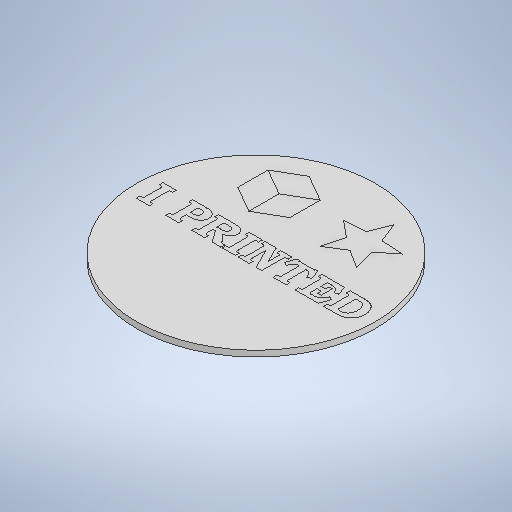
# Autodesk Inventor part: I_Printed
Saved by Autodesk Inventor 2025 (Build 290162000, 162)
## iProperties
Created: 2024-07-08
Part Number: I_Printed
Material: Generic
Document SubType Name: Modeling
Designer: ethan
Density: 1 g/cm^3
Appearance: Default
Author: ethan
Autodesk Inventor part; units mm, degrees
(part 1 of 2)
ref_plane "YZ Plane" through (0, 0, 0) normal (1, 0, 0) x (0, 1, 0)
ref_plane "XZ Plane" through (0, 0, 0) normal (0, 1, 0) x (-1, 0, 0)
ref_plane "XY Plane" through (0, 0, 0) normal (0, 0, 1) x (1, 0, 0)
sketch "Sketch2" plane through (0, 0, 0) normal (0, 1, 0) x (-1, 0, 0)
  circle A0 centre (0, 0) radius 50.8
  dimension "d2" = 101.6
  constraints: 1 centre point, 1 coincident
  measures "d2" diameter of A0
extrude "Extrusion1" add sketch "Sketch2" along normal blind 2.54
sketch "Sketch3" plane through (0, 2.54, 0) normal (0, 1, 0) x (1, 0, 0)
  line L0 (-46.0267, 6.3644) -> (46.9491, 6.3644) construction
  line L1 (46.9491, 6.3644) -> (46.9491, -11.3453) construction
  line L2 (46.9491, -11.3453) -> (-46.0267, -11.3453) construction
  line L3 (-46.0267, -11.3453) -> (-46.0267, 6.3644) construction
  line L4 (-45.4605, 5.9805) -> (-39.8942, 5.9805)
  line L5 (-39.8942, 5.9805) -> (-39.8942, 4.397)
  line L6 (-39.8942, 4.397) -> (-40.4028, 4.397)
  spline S0 degree 2 poles (-40.4028, 4.397) (-40.8443, 4.397) (-41.1322, 4.2435) (-41.2666, 3.9076) (-41.2666, 3.4277) knots 0 0 0 1 2 3 3 3
  line L7 (-41.2666, 3.4277) -> (-41.2666, -2.8871)
  spline S1 degree 2 poles (-41.2666, -2.8871) (-41.2666, -3.4053) (-41.1514, -3.7028) (-41.0171, -3.77) knots 0 0 0 1 2 2 2
  spline S2 degree 2 poles (-41.0171, -3.77) (-40.8443, -3.866) (-40.4988, -3.866) knots 0 0 0 1 1 1
  line L8 (-40.4988, -3.866) -> (-39.8942, -3.866)
  line L9 (-39.8942, -3.866) -> (-39.8942, -5.4495)
  line L10 (-39.8942, -5.4495) -> (-45.4605, -5.4495)
  line L11 (-45.4605, -5.4495) -> (-45.4605, -3.866)
  line L12 (-45.4605, -3.866) -> (-45.0094, -3.866)
  spline S3 degree 2 poles (-45.0094, -3.866) (-44.52, -3.866) (-44.232, -3.722) (-44.0881, -3.4245) (-44.0881, -2.9734) knots 0 0 0 1 2 3 3 3
  line L13 (-44.0881, -2.9734) -> (-44.0881, 3.3702)
  spline S4 degree 2 poles (-44.0881, 3.3702) (-44.0881, 3.9076) (-44.232, 4.2435) (-44.3952, 4.3299) knots 0 0 0 1 2 2 2
  spline S5 degree 2 poles (-44.3952, 4.3299) (-44.5104, 4.397) (-44.9518, 4.397) knots 0 0 0 1 1 1
  line L14 (-44.9518, 4.397) -> (-45.4605, 4.397)
  line L15 (-45.4605, 4.397) -> (-45.4605, 5.9805)
  line L16 (-32.946, 5.9805) -> (-26.9095, 5.9805)
  spline S6 degree 2 poles (-26.9095, 5.9805) (-25.7675, 5.9805) (-24.2511, 5.5103) (-23.1571, 4.5602) (-22.5717, 3.2646) (-22.5717, 2.5352) knots 0 0 0 1 2 3 4 4 4
  spline S7 degree 2 poles (-22.5717, 2.5352) (-22.5717, 1.0669) (-24.827, -0.9197) (-26.8039, -0.9197) knots 0 0 0 1 2 2 2
  line L17 (-26.8039, -0.9197) -> (-28.7521, -0.9197)
  line L18 (-28.7521, -0.9197) -> (-28.7521, -3.0598)
  spline S8 degree 2 poles (-28.7521, -3.0598) (-28.7521, -3.4533) (-28.6945, -3.5589) knots 0 0 0 1 1 1
  spline S9 degree 2 poles (-28.6945, -3.5589) (-28.6178, -3.722) (-28.3203, -3.866) (-27.9556, -3.866) knots 0 0 0 1 2 2 2
  line L19 (-27.9556, -3.866) -> (-27.3797, -3.866)
  line L20 (-27.3797, -3.866) -> (-27.3797, -5.4495)
  line L21 (-27.3797, -5.4495) -> (-32.946, -5.4495)
  line L22 (-32.946, -5.4495) -> (-32.946, -3.866)
  line L23 (-32.946, -3.866) -> (-32.5621, -3.866)
  spline S10 degree 2 poles (-32.5621, -3.866) (-32.0535, -3.866) (-31.7176, -3.722) (-31.5736, -3.3957) (-31.5736, -2.8967) knots 0 0 0 1 2 3 3 3
  line L24 (-31.5736, -2.8967) -> (-31.5736, 3.3798)
  spline S11 degree 2 poles (-31.5736, 3.3798) (-31.5736, 3.9076) (-31.708, 4.2435) (-31.9959, 4.397) (-32.399, 4.397) knots 0 0 0 1 2 3 3 3
  line L25 (-32.399, 4.397) -> (-32.946, 4.397)
  line L26 (-32.946, 4.397) -> (-32.946, 5.9805)
  line L27 (-28.7521, 4.1091) -> (-28.7521, 0.8653)
  line L28 (-28.7521, 0.8653) -> (-27.7828, 0.8653)
  spline S12 degree 2 poles (-27.7828, 0.8653) (-26.8903, 0.8653) (-26.0554, 1.23) (-25.5467, 1.9978) (-25.5467, 2.516) knots 0 0 0 1 2 3 3 3
  spline S13 degree 2 poles (-25.5467, 2.516) (-25.5467, 3.303) (-26.1513, 3.7636) knots 0 0 0 1 1 1
  spline S14 degree 2 poles (-26.1513, 3.7636) (-26.6024, 4.1091) (-27.4853, 4.1091) knots 0 0 0 1 1 1
  line L29 (-27.4853, 4.1091) -> (-28.7521, 4.1091)
  line L30 (-21.9383, 5.9805) -> (-14.8941, 5.9805)
  spline S15 degree 2 poles (-14.8941, 5.9805) (-14.2127, 5.9805) (-12.6004, 5.731) (-11.2952, 4.8961) (-10.5754, 3.6197) (-10.5754, 2.8135) knots 0 0 0 1 2 3 4 4 4
  spline S16 degree 2 poles (-10.5754, 2.8135) (-10.5754, 1.5179) (-12.4373, -0.104) (-13.7041, -0.3439) knots 0 0 0 1 2 2 2
  line L31 (-13.7041, -0.3439) -> (-11.3528, -3.079)
  line L32 (-11.3528, -3.079) -> (-11.2568, -3.2038)
  spline S17 degree 2 poles (-11.2568, -3.2038) (-11.0265, -3.4821) (-10.6426, -3.7508) (-10.2683, -3.866) (-9.9324, -3.866) knots 0 0 0 1 2 3 3 3
  line L33 (-9.9324, -3.866) -> (-9.443, -3.866)
  line L34 (-9.443, -3.866) -> (-9.443, -5.4495)
  line L35 (-9.443, -5.4495) -> (-13.109, -5.4495)
  line L36 (-13.109, -5.4495) -> (-16.7751, -0.5262)
  line L37 (-16.7751, -0.5262) -> (-17.7252, -0.5262)
  line L38 (-17.7252, -0.5262) -> (-17.7252, -2.8007)
  spline S18 degree 2 poles (-17.7252, -2.8007) (-17.7252, -3.3957) (-17.5908, -3.7124) (-17.3125, -3.866) (-16.8711, -3.866) knots 0 0 0 1 2 3 3 3
  line L39 (-16.8711, -3.866) -> (-16.3528, -3.866)
  line L40 (-16.3528, -3.866) -> (-16.3528, -5.4495)
  line L41 (-16.3528, -5.4495) -> (-21.9383, -5.4495)
  line L42 (-21.9383, -5.4495) -> (-21.9383, -3.866)
  line L43 (-21.9383, -3.866) -> (-21.4296, -3.866)
  spline S19 degree 2 poles (-21.4296, -3.866) (-21.0266, -3.866) (-20.6907, -3.6932) (-20.6043, -3.5205) knots 0 0 0 1 2 2 2
  spline S20 degree 2 poles (-20.6043, -3.5205) (-20.5659, -3.4245) (-20.5659, -2.9063) knots 0 0 0 1 1 1
  line L44 (-20.5659, -2.9063) -> (-20.5659, 3.5237)
  spline S21 degree 2 poles (-20.5659, 3.5237) (-20.5659, 3.898) (-20.6907, 4.2147) (-20.825, 4.2627) knots 0 0 0 1 2 2 2
  spline S22 degree 2 poles (-20.825, 4.2627) (-21.0266, 4.3586) (-21.2761, 4.3586) knots 0 0 0 1 1 1
  line L45 (-21.2761, 4.3586) -> (-21.5064, 4.349)
  line L46 (-21.5064, 4.349) -> (-21.9383, 4.349)
  line L47 (-21.9383, 4.349) -> (-21.9383, 5.9805)
  line L48 (-17.7252, 4.0995) -> (-17.7252, 1.1437)
  line L49 (-17.7252, 1.1437) -> (-16.0265, 1.1437)
  spline S23 degree 2 poles (-16.0265, 1.1437) (-15.0284, 1.1437) (-14.04, 1.5083) (-13.5409, 2.1993) (-13.5409, 2.6888) knots 0 0 0 1 2 3 3 3
  spline S24 degree 2 poles (-13.5409, 2.6888) (-13.5409, 3.1398) (-14.0112, 3.7924) (-14.8653, 4.0995) (-15.8442, 4.0995) knots 0 0 0 1 2 3 3 3
  line L50 (-15.8442, 4.0995) -> (-17.7252, 4.0995)
  line L51 (-8.896, 5.9805) -> (-3.3297, 5.9805)
  line L52 (-3.3297, 5.9805) -> (-3.3297, 4.397)
  line L53 (-3.3297, 4.397) -> (-3.8384, 4.397)
  spline S25 degree 2 poles (-3.8384, 4.397) (-4.2798, 4.397) (-4.5677, 4.2435) (-4.7021, 3.9076) (-4.7021, 3.4277) knots 0 0 0 1 2 3 3 3
  line L54 (-4.7021, 3.4277) -> (-4.7021, -2.8871)
  spline S26 degree 2 poles (-4.7021, -2.8871) (-4.7021, -3.4053) (-4.5869, -3.7028) (-4.4526, -3.77) knots 0 0 0 1 2 2 2
  spline S27 degree 2 poles (-4.4526, -3.77) (-4.2798, -3.866) (-3.9343, -3.866) knots 0 0 0 1 1 1
  line L55 (-3.9343, -3.866) -> (-3.3297, -3.866)
  line L56 (-3.3297, -3.866) -> (-3.3297, -5.4495)
  line L57 (-3.3297, -5.4495) -> (-8.896, -5.4495)
  line L58 (-8.896, -5.4495) -> (-8.896, -3.866)
  line L59 (-8.896, -3.866) -> (-8.4449, -3.866)
  spline S28 degree 2 poles (-8.4449, -3.866) (-7.9555, -3.866) (-7.6676, -3.722) (-7.5236, -3.4245) (-7.5236, -2.9734) knots 0 0 0 1 2 3 3 3
  line L60 (-7.5236, -2.9734) -> (-7.5236, 3.3702)
  spline S29 degree 2 poles (-7.5236, 3.3702) (-7.5236, 3.9076) (-7.6676, 4.2435) (-7.8307, 4.3299) knots 0 0 0 1 2 2 2
  spline S30 degree 2 poles (-7.8307, 4.3299) (-7.9459, 4.397) (-8.3873, 4.397) knots 0 0 0 1 1 1
  line L61 (-8.3873, 4.397) -> (-8.896, 4.397)
  line L62 (-8.896, 4.397) -> (-8.896, 5.9805)
  line L63 (-2.1013, 5.9805) -> (2.5244, 5.9805)
  line L64 (2.5244, 5.9805) -> (5.8834, -0.6894)
  line L65 (5.8834, -0.6894) -> (5.8834, 3.3893)
  spline S31 degree 2 poles (5.8834, 3.3893) (5.8834, 3.9172) (5.8258, 4.0419) knots 0 0 0 1 1 1
  spline S32 degree 2 poles (5.8258, 4.0419) (5.749, 4.2435) (5.4707, 4.397) (5.0676, 4.397) knots 0 0 0 1 2 2 2
  line L66 (5.0676, 4.397) -> (4.511, 4.397)
  line L67 (4.511, 4.397) -> (4.511, 5.9805)
  line L68 (4.511, 5.9805) -> (9.2135, 5.9805)
  line L69 (9.2135, 5.9805) -> (9.2135, 4.397)
  line L70 (9.2135, 4.397) -> (8.6953, 4.397)
  spline S33 degree 2 poles (8.6953, 4.397) (8.3018, 4.397) (7.9755, 4.2147) (7.8412, 3.9076) (7.8412, 3.3893) knots 0 0 0 1 2 3 3 3
  line L71 (7.8412, 3.3893) -> (7.8412, -5.4495)
  line L72 (7.8412, -5.4495) -> (5.4899, -5.4495)
  line L73 (5.4899, -5.4495) -> (1.248, 2.9767)
  line L74 (1.248, 2.9767) -> (1.248, -2.9159)
  spline S34 degree 2 poles (1.248, -2.9159) (1.248, -3.4245) (1.3728, -3.7028) (1.6895, -3.866) (2.0734, -3.866) knots 0 0 0 1 2 3 3 3
  line L75 (2.0734, -3.866) -> (2.6204, -3.866)
  line L76 (2.6204, -3.866) -> (2.6204, -5.4495)
  line L77 (2.6204, -5.4495) -> (-2.1013, -5.4495)
  line L78 (-2.1013, -5.4495) -> (-2.1013, -3.866)
  line L79 (-2.1013, -3.866) -> (-1.6119, -3.866)
  spline S35 degree 2 poles (-1.6119, -3.866) (-1.2088, -3.866) (-0.9113, -3.722) (-0.7289, -3.3861) (-0.7289, -3.0406) knots 0 0 0 1 2 3 3 3
  line L80 (-0.7289, -3.0406) -> (-0.7289, 3.5141)
  spline S36 degree 2 poles (-0.7289, 3.5141) (-0.7289, 3.8884) (-0.8921, 4.2435) (-1.1704, 4.397) (-1.4967, 4.397) knots 0 0 0 1 2 3 3 3
  line L81 (-1.4967, 4.397) -> (-2.1013, 4.397)
  line L82 (-2.1013, 4.397) -> (-2.1013, 5.9805)
  line L83 (11.0849, 6.3644) -> (12.1598, 6.3644)
  line L84 (12.1598, 6.3644) -> (12.275, 5.9805)
  line L85 (12.275, 5.9805) -> (18.7241, 5.9805)
  line L86 (18.7241, 5.9805) -> (18.8585, 6.3644)
  line L87 (18.8585, 6.3644) -> (19.9429, 6.3644)
  line L88 (19.9429, 6.3644) -> (21.3633, 2.3529)
  line L89 (21.3633, 2.3529) -> (19.8374, 1.825)
  spline S37 degree 2 poles (19.8374, 1.825) (19.3287, 2.8231) (19.108, 3.1302) knots 0 0 0 1 1 1
  spline S38 degree 2 poles (19.108, 3.1302) (18.6761, 3.7252) (18.1099, 4.0707) knots 0 0 0 1 1 1
  spline S39 degree 2 poles (18.1099, 4.0707) (17.6877, 4.3299) (17.2654, 4.3299) knots 0 0 0 1 1 1
  spline S40 degree 2 poles (17.2654, 4.3299) (17.0639, 4.3299) (16.9199, 4.1379) (16.9199, 3.802) knots 0 0 0 1 2 2 2
  line L90 (16.9199, 3.802) -> (16.9199, -2.7623)
  spline S41 degree 2 poles (16.9199, -2.7623) (16.9199, -3.3381) (17.0063, -3.6356) (17.1982, -3.8084) (17.5437, -3.866) (18.2923, -3.866) knots 0 0 0 1 2 3 4 4 4
  line L91 (18.2923, -3.866) -> (18.2923, -5.4495)
  line L92 (18.2923, -5.4495) -> (12.726, -5.4495)
  line L93 (12.726, -5.4495) -> (12.726, -3.866)
  line L94 (12.726, -3.866) -> (13.0619, -3.866)
  spline S42 degree 2 poles (13.0619, -3.866) (13.6185, -3.866) (13.9352, -3.722) (14.0984, -3.3765) (14.0984, -2.8199) knots 0 0 0 1 2 3 3 3
  line L95 (14.0984, -2.8199) -> (14.0984, 3.898)
  spline S43 degree 2 poles (14.0984, 3.898) (14.0984, 4.1859) (13.964, 4.3299) (13.7529, 4.3299) knots 0 0 0 1 2 2 2
  spline S44 degree 2 poles (13.7529, 4.3299) (13.3306, 4.3299) (12.275, 3.6869) (11.8719, 3.111) knots 0 0 0 1 2 2 2
  spline S45 degree 2 poles (11.8719, 3.111) (11.6991, 2.8807) (11.1713, 1.825) knots 0 0 0 1 1 1
  line L96 (11.1713, 1.825) -> (9.6742, 2.3529)
  line L97 (9.6742, 2.3529) -> (11.0849, 6.3644)
  line L98 (22.0447, 5.9805) -> (31.5841, 5.9805)
  line L99 (31.5841, 5.9805) -> (32.8893, 2.3625)
  line L100 (32.8893, 2.3625) -> (31.4017, 1.825)
  spline S46 degree 2 poles (31.4017, 1.825) (31.0275, 2.7176) (30.0198, 3.7924) (28.801, 4.1475) (27.9852, 4.1475) knots 0 0 0 1 2 3 3 3
  line L101 (27.9852, 4.1475) -> (26.2386, 4.1475)
  line L102 (26.2386, 4.1475) -> (26.2386, 1.2972)
  line L103 (26.2386, 1.2972) -> (26.8144, 1.2972)
  spline S47 degree 2 poles (26.8144, 1.2972) (27.4574, 1.2972) (27.9084, 1.4891) (28.11, 1.8826) (28.11, 2.4872) knots 0 0 0 1 2 3 3 3
  line L104 (28.11, 2.4872) -> (28.11, 2.9191)
  line L105 (28.11, 2.9191) -> (29.5687, 2.9191)
  line L106 (29.5687, 2.9191) -> (29.5687, -1.9178)
  line L107 (29.5687, -1.9178) -> (28.11, -1.9178)
  line L108 (28.11, -1.9178) -> (28.11, -1.4283)
  spline S48 degree 2 poles (28.11, -1.4283) (28.11, -0.9197) (27.87, -0.459) (27.4574, -0.2959) (26.7568, -0.2959) knots 0 0 0 1 2 3 3 3
  line L109 (26.7568, -0.2959) -> (26.2386, -0.2959)
  line L110 (26.2386, -0.2959) -> (26.2386, -2.9159)
  spline S49 degree 2 poles (26.2386, -2.9159) (26.2386, -3.3381) (26.3249, -3.5205) (26.5553, -3.6164) (26.9487, -3.6164) knots 0 0 0 1 2 3 3 3
  line L111 (26.9487, -3.6164) -> (27.9084, -3.6164)
  spline S50 degree 2 poles (27.9084, -3.6164) (28.9833, -3.6164) (30.4612, -3.0022) (31.6225, -1.6299) (31.9296, -0.6894) knots 0 0 0 1 2 3 3 3
  line L112 (31.9296, -0.6894) -> (33.4267, -1.198)
  line L113 (33.4267, -1.198) -> (31.9296, -5.4495)
  line L114 (31.9296, -5.4495) -> (22.0447, -5.4495)
  line L115 (22.0447, -5.4495) -> (22.0447, -3.866)
  line L116 (22.0447, -3.866) -> (22.3326, -3.866)
  spline S51 degree 2 poles (22.3326, -3.866) (22.8988, -3.866) (23.2923, -3.7028) (23.3787, -3.5013) knots 0 0 0 1 2 2 2
  spline S52 degree 2 poles (23.3787, -3.5013) (23.4171, -3.3765) (23.4171, -2.8007) knots 0 0 0 1 1 1
  line L117 (23.4171, -2.8007) -> (23.4171, 3.4181)
  spline S53 degree 2 poles (23.4171, 3.4181) (23.4171, 3.9268) (23.2827, 4.2435) (22.9852, 4.397) (22.5533, 4.397) knots 0 0 0 1 2 3 3 3
  line L118 (22.5533, 4.397) -> (22.0447, 4.397)
  line L119 (22.0447, 4.397) -> (22.0447, 5.9805)
  line L120 (34.0985, 5.9805) -> (40.087, 5.9805)
  spline S54 degree 2 poles (40.087, 5.9805) (42.1312, 5.9805) (44.54, 4.6849) (45.9699, 2.1417) (45.9699, 0.3663) knots 0 0 0 1 2 3 3 3
  spline S55 degree 2 poles (45.9699, 0.3663) (45.9699, -0.8717) (45.2406, -2.8199) (43.801, -4.3842) (42.9757, -4.7777) knots 0 0 0 1 2 3 3 3
  spline S56 degree 2 poles (42.9757, -4.7777) (42.3519, -5.0752) (40.0582, -5.4495) (39.3768, -5.4495) knots 0 0 0 1 2 2 2
  line L121 (39.3768, -5.4495) -> (34.0985, -5.4495)
  line L122 (34.0985, -5.4495) -> (34.0985, -3.866)
  line L123 (34.0985, -3.866) -> (34.492, -3.866)
  spline S57 degree 2 poles (34.492, -3.866) (34.991, -3.866) (35.3077, -3.7028) (35.4037, -3.5013) knots 0 0 0 1 2 2 2
  spline S58 degree 2 poles (35.4037, -3.5013) (35.4709, -3.3477) (35.4709, -2.8295) knots 0 0 0 1 1 1
  line L124 (35.4709, -2.8295) -> (35.4709, 3.4181)
  spline S59 degree 2 poles (35.4709, 3.4181) (35.4709, 3.9364) (35.3269, 4.2435) (35.0102, 4.397) (34.492, 4.397) knots 0 0 0 1 2 3 3 3
  line L125 (34.492, 4.397) -> (34.0985, 4.397)
  line L126 (34.0985, 4.397) -> (34.0985, 5.9805)
  line L127 (38.2828, 4.1475) -> (38.2828, -2.9639)
  spline S60 degree 2 poles (38.2828, -2.9639) (38.2828, -3.3189) (38.3212, -3.4053) knots 0 0 0 1 1 1
  spline S61 degree 2 poles (38.3212, -3.4053) (38.3883, -3.5301) (38.6475, -3.6164) (39.1273, -3.6164) knots 0 0 0 1 2 2 2
  spline S62 degree 2 poles (39.1273, -3.6164) (40.4709, -3.6164) (41.9872, -2.7911) (42.9181, -0.9581) (42.9181, 0.2991) knots 0 0 0 1 2 3 3 3
  spline S63 degree 2 poles (42.9181, 0.2991) (42.9181, 1.5467) (42.0448, 3.3893) (40.7492, 4.1475) (39.54, 4.1475) knots 0 0 0 1 2 3 3 3
  line L128 (39.54, 4.1475) -> (38.2828, 4.1475)
  point P0 (0, 0)
  constraints: 2 other
extrude "Extrusion2" cut sketch "Sketch3" against normal blind 10.4775
sketch "Sketch4" plane through (0, 2.54, 0) normal (0, 1, 0) x (1, 0, 0)
  circle A0 centre (0, 0) radius 50.8 projected
  line L0 (22.0447, 4.397) -> (22.0447, 5.9805) projected
  line L1 (22.0447, 5.9805) -> (31.5841, 5.9805) projected
  line L2 (31.5841, 5.9805) -> (32.8893, 2.3625) projected
  line L3 (32.8893, 2.3625) -> (31.4017, 1.825) projected
  spline S0 degree 2 poles (31.4017, 1.825) (31.0275, 2.7176) (30.0198, 3.7924) (28.801, 4.1475) (27.9852, 4.1475) knots 0 0 0 0.333333 0.666667 1 1 1 projected
  line L4 (27.9852, 4.1475) -> (26.2386, 4.1475) projected
  line L5 (26.2386, 4.1475) -> (26.2386, 1.2972) projected
  line L6 (26.2386, 1.2972) -> (26.8144, 1.2972) projected
  spline S1 degree 2 poles (26.8144, 1.2972) (27.4574, 1.2972) (27.9084, 1.4891) (28.11, 1.8826) (28.11, 2.4872) knots 0 0 0 0.333333 0.666667 1 1 1 projected
  line L7 (28.11, 2.4872) -> (28.11, 2.9191) projected
  line L8 (28.11, 2.9191) -> (29.5687, 2.9191) projected
  line L9 (29.5687, 2.9191) -> (29.5687, -1.9178) projected
  line L10 (29.5687, -1.9178) -> (28.11, -1.9178) projected
  line L11 (28.11, -1.9178) -> (28.11, -1.4283) projected
  spline S2 degree 2 poles (28.11, -1.4283) (28.11, -0.9197) (27.87, -0.459) (27.4574, -0.2959) (26.7568, -0.2959) knots 0 0 0 0.333333 0.666667 1 1 1 projected
  line L12 (26.7568, -0.2959) -> (26.2386, -0.2959) projected
  line L13 (26.2386, -0.2959) -> (26.2386, -2.9159) projected
  spline S3 degree 2 poles (26.2386, -2.9159) (26.2386, -3.3381) (26.3249, -3.5205) (26.5553, -3.6164) (26.9487, -3.6164) knots 0 0 0 0.333333 0.666667 1 1 1 projected
  line L14 (26.9487, -3.6164) -> (27.9084, -3.6164) projected
  spline S4 degree 2 poles (27.9084, -3.6164) (28.9833, -3.6164) (30.4612, -3.0022) (31.6225, -1.6299) (31.9296, -0.6894) knots 0 0 0 0.333333 0.666667 1 1 1 projected
  line L15 (31.9296, -0.6894) -> (33.4267, -1.198) projected
  line L16 (33.4267, -1.198) -> (31.9296, -5.4495) projected
  line L17 (31.9296, -5.4495) -> (22.0447, -5.4495) projected
  line L18 (22.0447, -5.4495) -> (22.0447, -3.866) projected
  line L19 (22.0447, -3.866) -> (22.3326, -3.866) projected
  spline S5 degree 2 poles (22.3326, -3.866) (22.8988, -3.866) (23.2923, -3.7028) (23.3787, -3.5013) knots 0 0 0 0.5 1 1 1 projected
  spline S6 degree 2 poles (23.3787, -3.5013) (23.4171, -3.3765) (23.4171, -2.8007) knots 0 0 0 1 1 1 projected
  line L20 (23.4171, -2.8007) -> (23.4171, 3.4181) projected
  spline S7 degree 2 poles (23.4171, 3.4181) (23.4171, 3.9268) (23.2827, 4.2435) (22.9852, 4.397) (22.5533, 4.397) knots 0 0 0 0.333333 0.666667 1 1 1 projected
  line L21 (22.5533, 4.397) -> (22.0447, 4.397) projected
  line L22 (-2.1013, 4.397) -> (-2.1013, 5.9805) projected
  line L23 (-2.1013, 5.9805) -> (2.5244, 5.9805) projected
  line L24 (2.5244, 5.9805) -> (5.8834, -0.6894) projected
  line L25 (5.8834, -0.6894) -> (5.8834, 3.3893) projected
  spline S8 degree 2 poles (5.8834, 3.3893) (5.8834, 3.9172) (5.8258, 4.0419) knots 0 0 0 1 1 1 projected
  spline S9 degree 2 poles (5.8258, 4.0419) (5.749, 4.2435) (5.4707, 4.397) (5.0676, 4.397) knots 0 0 0 0.5 1 1 1 projected
  line L26 (5.0676, 4.397) -> (4.511, 4.397) projected
  line L27 (4.511, 4.397) -> (4.511, 5.9805) projected
  line L28 (4.511, 5.9805) -> (9.2135, 5.9805) projected
  line L29 (9.2135, 5.9805) -> (9.2135, 4.397) projected
  line L30 (9.2135, 4.397) -> (8.6953, 4.397) projected
  spline S10 degree 2 poles (8.6953, 4.397) (8.3018, 4.397) (7.9755, 4.2147) (7.8412, 3.9076) (7.8412, 3.3893) knots 0 0 0 0.333333 0.666667 1 1 1 projected
  line L31 (7.8412, 3.3893) -> (7.8412, -5.4495) projected
  line L32 (7.8412, -5.4495) -> (5.4899, -5.4495) projected
  line L33 (5.4899, -5.4495) -> (1.248, 2.9767) projected
  line L34 (1.248, 2.9767) -> (1.248, -2.9159) projected
  spline S11 degree 2 poles (1.248, -2.9159) (1.248, -3.4245) (1.3728, -3.7028) (1.6895, -3.866) (2.0734, -3.866) knots 0 0 0 0.333333 0.666667 1 1 1 projected
  line L35 (2.0734, -3.866) -> (2.6204, -3.866) projected
  line L36 (2.6204, -3.866) -> (2.6204, -5.4495) projected
  line L37 (2.6204, -5.4495) -> (-2.1013, -5.4495) projected
  line L38 (-2.1013, -5.4495) -> (-2.1013, -3.866) projected
  line L39 (-2.1013, -3.866) -> (-1.6119, -3.866) projected
  spline S12 degree 2 poles (-1.6119, -3.866) (-1.2088, -3.866) (-0.9113, -3.722) (-0.7289, -3.3861) (-0.7289, -3.0406) knots 0 0 0 0.333333 0.666667 1 1 1 projected
  line L40 (-0.7289, -3.0406) -> (-0.7289, 3.5141) projected
  spline S13 degree 2 poles (-0.7289, 3.5141) (-0.7289, 3.8884) (-0.8921, 4.2435) (-1.1704, 4.397) (-1.4967, 4.397) knots 0 0 0 0.333333 0.666667 1 1 1 projected
  line L41 (-1.4967, 4.397) -> (-2.1013, 4.397) projected
  line L42 (-45.4605, 4.397) -> (-45.4605, 5.9805) projected
  line L43 (-45.4605, 5.9805) -> (-39.8942, 5.9805) projected
  line L44 (-39.8942, 5.9805) -> (-39.8942, 4.397) projected
  line L45 (-39.8942, 4.397) -> (-40.4028, 4.397) projected
  spline S14 degree 2 poles (-40.4028, 4.397) (-40.8443, 4.397) (-41.1322, 4.2435) (-41.2666, 3.9076) (-41.2666, 3.4277) knots 0 0 0 0.333333 0.666667 1 1 1 projected
  line L46 (-41.2666, 3.4277) -> (-41.2666, -2.8871) projected
  spline S15 degree 2 poles (-41.2666, -2.8871) (-41.2666, -3.4053) (-41.1514, -3.7028) (-41.0171, -3.77) knots 0 0 0 0.5 1 1 1 projected
  spline S16 degree 2 poles (-41.0171, -3.77) (-40.8443, -3.866) (-40.4988, -3.866) knots 0 0 0 1 1 1 projected
  line L47 (-40.4988, -3.866) -> (-39.8942, -3.866) projected
  line L48 (-39.8942, -3.866) -> (-39.8942, -5.4495) projected
  line L49 (-39.8942, -5.4495) -> (-45.4605, -5.4495) projected
  line L50 (-45.4605, -5.4495) -> (-45.4605, -3.866) projected
  line L51 (-45.4605, -3.866) -> (-45.0094, -3.866) projected
  spline S17 degree 2 poles (-45.0094, -3.866) (-44.52, -3.866) (-44.232, -3.722) (-44.0881, -3.4245) (-44.0881, -2.9734) knots 0 0 0 0.333333 0.666667 1 1 1 projected
  line L52 (-44.0881, -2.9734) -> (-44.0881, 3.3702) projected
  spline S18 degree 2 poles (-44.0881, 3.3702) (-44.0881, 3.9076) (-44.232, 4.2435) (-44.3952, 4.3299) knots 0 0 0 0.5 1 1 1 projected
  spline S19 degree 2 poles (-44.3952, 4.3299) (-44.5104, 4.397) (-44.9518, 4.397) knots 0 0 0 1 1 1 projected
  line L53 (-44.9518, 4.397) -> (-45.4605, 4.397) projected
  line L54 (-32.946, 4.397) -> (-32.946, 5.9805) projected
  line L55 (-32.946, 5.9805) -> (-26.9095, 5.9805) projected
  spline S20 degree 2 poles (-26.9095, 5.9805) (-25.7675, 5.9805) (-24.2511, 5.5103) (-23.1571, 4.5602) (-22.5717, 3.2646) (-22.5717, 2.5352) knots 0 0 0 0.25 0.5 0.75 1 1 1 projected
  spline S21 degree 2 poles (-22.5717, 2.5352) (-22.5717, 1.0669) (-24.827, -0.9197) (-26.8039, -0.9197) knots 0 0 0 0.5 1 1 1 projected
  line L56 (-26.8039, -0.9197) -> (-28.7521, -0.9197) projected
  line L57 (-28.7521, -0.9197) -> (-28.7521, -3.0598) projected
  spline S22 degree 2 poles (-28.7521, -3.0598) (-28.7521, -3.4533) (-28.6945, -3.5589) knots 0 0 0 1 1 1 projected
  spline S23 degree 2 poles (-28.6945, -3.5589) (-28.6178, -3.722) (-28.3203, -3.866) (-27.9556, -3.866) knots 0 0 0 0.5 1 1 1 projected
  line L58 (-27.9556, -3.866) -> (-27.3797, -3.866) projected
  line L59 (-27.3797, -3.866) -> (-27.3797, -5.4495) projected
  line L60 (-27.3797, -5.4495) -> (-32.946, -5.4495) projected
  line L61 (-32.946, -5.4495) -> (-32.946, -3.866) projected
  line L62 (-32.946, -3.866) -> (-32.5621, -3.866) projected
  spline S24 degree 2 poles (-32.5621, -3.866) (-32.0535, -3.866) (-31.7176, -3.722) (-31.5736, -3.3957) (-31.5736, -2.8967) knots 0 0 0 0.333333 0.666667 1 1 1 projected
  line L63 (-31.5736, -2.8967) -> (-31.5736, 3.3798) projected
  spline S25 degree 2 poles (-31.5736, 3.3798) (-31.5736, 3.9076) (-31.708, 4.2435) (-31.9959, 4.397) (-32.399, 4.397) knots 0 0 0 0.333333 0.666667 1 1 1 projected
  line L64 (-32.399, 4.397) -> (-32.946, 4.397) projected
  line L65 (-21.9383, 4.349) -> (-21.9383, 5.9805) projected
  line L66 (-21.9383, 5.9805) -> (-14.8941, 5.9805) projected
  spline S26 degree 2 poles (-14.8941, 5.9805) (-14.2127, 5.9805) (-12.6004, 5.731) (-11.2952, 4.8961) (-10.5754, 3.6197) (-10.5754, 2.8135) knots 0 0 0 0.25 0.5 0.75 1 1 1 projected
  spline S27 degree 2 poles (-10.5754, 2.8135) (-10.5754, 1.5179) (-12.4373, -0.104) (-13.7041, -0.3439) knots 0 0 0 0.5 1 1 1 projected
  line L67 (-13.7041, -0.3439) -> (-11.3528, -3.079) projected
  line L68 (-11.3528, -3.079) -> (-11.2568, -3.2038) projected
  spline S28 degree 2 poles (-11.2568, -3.2038) (-11.0265, -3.4821) (-10.6426, -3.7508) (-10.2683, -3.866) (-9.9324, -3.866) knots 0 0 0 0.333333 0.666667 1 1 1 projected
  line L69 (-9.9324, -3.866) -> (-9.443, -3.866) projected
  line L70 (-9.443, -3.866) -> (-9.443, -5.4495) projected
  line L71 (-9.443, -5.4495) -> (-13.109, -5.4495) projected
  line L72 (-13.109, -5.4495) -> (-16.7751, -0.5262) projected
  line L73 (-16.7751, -0.5262) -> (-17.7252, -0.5262) projected
  line L74 (-17.7252, -0.5262) -> (-17.7252, -2.8007) projected
  spline S29 degree 2 poles (-17.7252, -2.8007) (-17.7252, -3.3957) (-17.5908, -3.7124) (-17.3125, -3.866) (-16.8711, -3.866) knots 0 0 0 0.333333 0.666667 1 1 1 projected
  line L75 (-16.8711, -3.866) -> (-16.3528, -3.866) projected
  line L76 (-16.3528, -3.866) -> (-16.3528, -5.4495) projected
  line L77 (-16.3528, -5.4495) -> (-21.9383, -5.4495) projected
  line L78 (-21.9383, -5.4495) -> (-21.9383, -3.866) projected
  line L79 (-21.9383, -3.866) -> (-21.4296, -3.866) projected
  spline S30 degree 2 poles (-21.4296, -3.866) (-21.0266, -3.866) (-20.6907, -3.6932) (-20.6043, -3.5205) knots 0 0 0 0.5 1 1 1 projected
  spline S31 degree 2 poles (-20.6043, -3.5205) (-20.5659, -3.4245) (-20.5659, -2.9063) knots 0 0 0 1 1 1 projected
  line L80 (-20.5659, -2.9063) -> (-20.5659, 3.5237) projected
  spline S32 degree 2 poles (-20.5659, 3.5237) (-20.5659, 3.898) (-20.6907, 4.2147) (-20.825, 4.2627) knots 0 0 0 0.5 1 1 1 projected
  spline S33 degree 2 poles (-20.825, 4.2627) (-21.0266, 4.3586) (-21.2761, 4.3586) knots 0 0 0 1 1 1 projected
  line L81 (-21.2761, 4.3586) -> (-21.5064, 4.349) projected
  line L82 (-21.5064, 4.349) -> (-21.9383, 4.349) projected
  line L83 (-8.896, 4.397) -> (-8.896, 5.9805) projected
  line L84 (-8.896, 5.9805) -> (-3.3297, 5.9805) projected
  line L85 (-3.3297, 5.9805) -> (-3.3297, 4.397) projected
  line L86 (-3.3297, 4.397) -> (-3.8384, 4.397) projected
  spline S34 degree 2 poles (-3.8384, 4.397) (-4.2798, 4.397) (-4.5677, 4.2435) (-4.7021, 3.9076) (-4.7021, 3.4277) knots 0 0 0 0.333333 0.666667 1 1 1 projected
  line L87 (-4.7021, 3.4277) -> (-4.7021, -2.8871) projected
  spline S35 degree 2 poles (-4.7021, -2.8871) (-4.7021, -3.4053) (-4.5869, -3.7028) (-4.4526, -3.77) knots 0 0 0 0.5 1 1 1 projected
  spline S36 degree 2 poles (-4.4526, -3.77) (-4.2798, -3.866) (-3.9343, -3.866) knots 0 0 0 1 1 1 projected
  line L88 (-3.9343, -3.866) -> (-3.3297, -3.866) projected
  line L89 (-3.3297, -3.866) -> (-3.3297, -5.4495) projected
  line L90 (-3.3297, -5.4495) -> (-8.896, -5.4495) projected
  line L91 (-8.896, -5.4495) -> (-8.896, -3.866) projected
  line L92 (-8.896, -3.866) -> (-8.4449, -3.866) projected
  spline S37 degree 2 poles (-8.4449, -3.866) (-7.9555, -3.866) (-7.6676, -3.722) (-7.5236, -3.4245) (-7.5236, -2.9734) knots 0 0 0 0.333333 0.666667 1 1 1 projected
  line L93 (-7.5236, -2.9734) -> (-7.5236, 3.3702) projected
  spline S38 degree 2 poles (-7.5236, 3.3702) (-7.5236, 3.9076) (-7.6676, 4.2435) (-7.8307, 4.3299) knots 0 0 0 0.5 1 1 1 projected
  spline S39 degree 2 poles (-7.8307, 4.3299) (-7.9459, 4.397) (-8.3873, 4.397) knots 0 0 0 1 1 1 projected
  line L94 (-8.3873, 4.397) -> (-8.896, 4.397) projected
  line L95 (9.6742, 2.3529) -> (11.0849, 6.3644) projected
  line L96 (11.0849, 6.3644) -> (12.1598, 6.3644) projected
  line L97 (12.1598, 6.3644) -> (12.275, 5.9805) projected
  line L98 (12.275, 5.9805) -> (18.7241, 5.9805) projected
  line L99 (18.7241, 5.9805) -> (18.8585, 6.3644) projected
  line L100 (18.8585, 6.3644) -> (19.9429, 6.3644) projected
  line L101 (19.9429, 6.3644) -> (21.3633, 2.3529) projected
  line L102 (21.3633, 2.3529) -> (19.8374, 1.825) projected
  spline S40 degree 2 poles (19.8374, 1.825) (19.3287, 2.8231) (19.108, 3.1302) knots 0 0 0 1 1 1 projected
  spline S41 degree 2 poles (19.108, 3.1302) (18.6761, 3.7252) (18.1099, 4.0707) knots 0 0 0 1 1 1 projected
  spline S42 degree 2 poles (18.1099, 4.0707) (17.6877, 4.3299) (17.2654, 4.3299) knots 0 0 0 1 1 1 projected
  spline S43 degree 2 poles (17.2654, 4.3299) (17.0639, 4.3299) (16.9199, 4.1379) (16.9199, 3.802) knots 0 0 0 0.5 1 1 1 projected
  line L103 (16.9199, 3.802) -> (16.9199, -2.7623) projected
  spline S44 degree 2 poles (16.9199, -2.7623) (16.9199, -3.3381) (17.0063, -3.6356) (17.1982, -3.8084) (17.5437, -3.866) (18.2923, -3.866) knots 0 0 0 0.25 0.5 0.75 1 1 1 projected
  line L104 (18.2923, -3.866) -> (18.2923, -5.4495) projected
  line L105 (18.2923, -5.4495) -> (12.726, -5.4495) projected
  line L106 (12.726, -5.4495) -> (12.726, -3.866) projected
  line L107 (12.726, -3.866) -> (13.0619, -3.866) projected
  spline S45 degree 2 poles (13.0619, -3.866) (13.6185, -3.866) (13.9352, -3.722) (14.0984, -3.3765) (14.0984, -2.8199) knots 0 0 0 0.333333 0.666667 1 1 1 projected
  line L108 (14.0984, -2.8199) -> (14.0984, 3.898) projected
  spline S46 degree 2 poles (14.0984, 3.898) (14.0984, 4.1859) (13.964, 4.3299) (13.7529, 4.3299) knots 0 0 0 0.5 1 1 1 projected
  spline S47 degree 2 poles (13.7529, 4.3299) (13.3306, 4.3299) (12.275, 3.6869) (11.8719, 3.111) knots 0 0 0 0.5 1 1 1 projected
  spline S48 degree 2 poles (11.8719, 3.111) (11.6991, 2.8807) (11.1713, 1.825) knots 0 0 0 1 1 1 projected
  line L109 (11.1713, 1.825) -> (9.6742, 2.3529) projected
  line L110 (34.0985, 4.397) -> (34.0985, 5.9805) projected
  line L111 (34.0985, 5.9805) -> (40.087, 5.9805) projected
  spline S49 degree 2 poles (40.087, 5.9805) (42.1312, 5.9805) (44.54, 4.6849) (45.9699, 2.1417) (45.9699, 0.3663) knots 0 0 0 0.333333 0.666667 1 1 1 projected
  spline S50 degree 2 poles (45.9699, 0.3663) (45.9699, -0.8717) (45.2406, -2.8199) (43.801, -4.3842) (42.9757, -4.7777) knots 0 0 0 0.333333 0.666667 1 1 1 projected
  spline S51 degree 2 poles (42.9757, -4.7777) (42.3519, -5.0752) (40.0582, -5.4495) (39.3768, -5.4495) knots 0 0 0 0.5 1 1 1 projected
  line L112 (39.3768, -5.4495) -> (34.0985, -5.4495) projected
  line L113 (34.0985, -5.4495) -> (34.0985, -3.866) projected
  line L114 (34.0985, -3.866) -> (34.492, -3.866) projected
  spline S52 degree 2 poles (34.492, -3.866) (34.991, -3.866) (35.3077, -3.7028) (35.4037, -3.5013) knots 0 0 0 0.5 1 1 1 projected
  spline S53 degree 2 poles (35.4037, -3.5013) (35.4709, -3.3477) (35.4709, -2.8295) knots 0 0 0 1 1 1 projected
  line L115 (35.4709, -2.8295) -> (35.4709, 3.4181) projected
  spline S54 degree 2 poles (35.4709, 3.4181) (35.4709, 3.9364) (35.3269, 4.2435) (35.0102, 4.397) (34.492, 4.397) knots 0 0 0 0.333333 0.666667 1 1 1 projected
  line L116 (34.492, 4.397) -> (34.0985, 4.397) projected
  line L117 (-28.7521, 0.8653) -> (-27.7828, 0.8653) projected
  spline S55 degree 2 poles (-27.7828, 0.8653) (-26.8903, 0.8653) (-26.0554, 1.23) (-25.5467, 1.9978) (-25.5467, 2.516) knots 0 0 0 0.333333 0.666667 1 1 1 projected
  spline S56 degree 2 poles (-25.5467, 2.516) (-25.5467, 3.303) (-26.1513, 3.7636) knots 0 0 0 1 1 1 projected
  spline S57 degree 2 poles (-26.1513, 3.7636) (-26.6024, 4.1091) (-27.4853, 4.1091) knots 0 0 0 1 1 1 projected
  line L118 (-27.4853, 4.1091) -> (-28.7521, 4.1091) projected
  line L119 (-28.7521, 4.1091) -> (-28.7521, 0.8653) projected
  line L120 (-17.7252, 1.1437) -> (-16.0265, 1.1437) projected
  spline S58 degree 2 poles (-16.0265, 1.1437) (-15.0284, 1.1437) (-14.04, 1.5083) (-13.5409, 2.1993) (-13.5409, 2.6888) knots 0 0 0 0.333333 0.666667 1 1 1 projected
  spline S59 degree 2 poles (-13.5409, 2.6888) (-13.5409, 3.1398) (-14.0112, 3.7924) (-14.8653, 4.0995) (-15.8442, 4.0995) knots 0 0 0 0.333333 0.666667 1 1 1 projected
  line L121 (-15.8442, 4.0995) -> (-17.7252, 4.0995) projected
  line L122 (-17.7252, 4.0995) -> (-17.7252, 1.1437) projected
  spline S60 degree 2 poles (38.2828, -2.9639) (38.2828, -3.3189) (38.3212, -3.4053) knots 0 0 0 1 1 1 projected
  spline S61 degree 2 poles (38.3212, -3.4053) (38.3883, -3.5301) (38.6475, -3.6164) (39.1273, -3.6164) knots 0 0 0 0.5 1 1 1 projected
  spline S62 degree 2 poles (39.1273, -3.6164) (40.4709, -3.6164) (41.9872, -2.7911) (42.9181, -0.9581) (42.9181, 0.2991) knots 0 0 0 0.333333 0.666667 1 1 1 projected
  spline S63 degree 2 poles (42.9181, 0.2991) (42.9181, 1.5467) (42.0448, 3.3893) (40.7492, 4.1475) (39.54, 4.1475) knots 0 0 0 0.333333 0.666667 1 1 1 projected
  line L123 (39.54, 4.1475) -> (38.2828, 4.1475) projected
  line L124 (38.2828, 4.1475) -> (38.2828, -2.9639) projected
  constraints: 64 other
extrude "Extrusion3" add sketch "Sketch4" against normal blind 2.54 separate body contours L0 L1 L2 L3 S0 L4 L5 L6 S1 L7 L8 L9 L10 L11 S2 L12 L13 S3 L14 S4 L15 L16 L17 L18 L19 S5 S6 L20 S7 L21 | L22 L23 L24 L25 S8 S9 L26 L27 L28 L29 L30 S10 L31 L32 L33 L34 S11 L35 L36 L37 L38 L39 S12 L40 S13 L41 | L42 L43 L44 L45 S14 L46 S15 S16 L47 L48 L49 L50 L51 S17 L52 S18 S19 L53 | L54 L55 S20 S21 L56 L57 S22 S23 L58 L59 L60 L61 L62 S24 L63 S25 L64 | L65 L66 S26 S27 L67 L68 S28 L69 L70 L71 L72 L73 L74 S29 L75 L76 L77 L78 L79 S30 S31 L80 S32 S33 L81 L82 | L83 L84 L85 L86 S34 L87 S35 S36 L88 L89 L90 L91 L92 S37 L93 S38 S39 L94 | L95 L96 L97 L98 L99 L100 L101 L102 S40 S41 S42 S43 L103 S44 L104 L105 L106 L107 S45 L108 S46 S47 S48 L109 | L110 L111 S49 S50 S51 L112 L113 L114 S52 S53 L115 S54 L116
sketch "Sketch5" plane through (0, 2.54, 0) normal (0, 1, 0) x (1, 0, 0)
  line L0 (-16.7308, 39.3139) -> (-5.6361, 32.9084)
  line L1 (-5.6361, 32.9084) -> (-5.6361, 20.0974)
  line L2 (-5.6361, 20.0974) -> (-16.7308, 13.6918)
  line L3 (-16.7308, 13.6918) -> (-27.8255, 20.0974)
  line L4 (-27.8255, 20.0974) -> (-27.8255, 32.9084)
  line L5 (-27.8255, 32.9084) -> (-16.7308, 39.3139)
  line L6 (22.4402, 31.1118) -> (19.0916, 39.5891)
  line L7 (22.4402, 31.1118) -> (31.5374, 30.5468)
  line L8 (24.5097, 24.7424) -> (31.5374, 30.5468)
  line L9 (24.5097, 24.7424) -> (26.7836, 15.9159)
  line L10 (26.7836, 15.9159) -> (19.0916, 20.806)
  line L11 (19.0916, 20.806) -> (11.3997, 15.9159)
  line L12 (13.6736, 24.7424) -> (11.3997, 15.9159)
  line L13 (13.6736, 24.7424) -> (6.6459, 30.5468)
  line L14 (15.7431, 31.1118) -> (6.6459, 30.5468)
  line L15 (15.7431, 31.1118) -> (19.0916, 39.5891)
  line L16 (6.6459, 30.5468) -> (8.6061, 31.9709)
  line L17 (17.1314, 38.165) -> (19.0916, 39.5891)
  line L18 (19.0916, 39.5891) -> (23.0914, 36.6832)
  line L19 (29.5772, 31.9709) -> (31.5374, 30.5468)
  line L20 (31.5374, 30.5468) -> (30.7887, 28.2424)
  line L21 (27.5323, 18.2202) -> (26.7836, 15.9159)
  line L22 (26.7836, 15.9159) -> (23.7959, 15.9159)
  line L23 (13.8227, 15.9159) -> (11.3997, 15.9159)
  line L24 (11.3997, 15.9159) -> (10.651, 18.2202)
  line L25 (8.5374, 24.7254) -> (6.6459, 30.5468)
  point P0 (0, 0)
  point P1 (-16.7308, 26.5029)
  point P2 (19.0916, 26.5029)
  point P3 (19.0916, 26.5029)
  constraints: 52 end point, 10 point on line, 2 horizontal, 1 coincident, 1 vertical, 25 other
extrude "Extrusion4" cut sketch "Sketch5" against normal blind 2.54 bodies 1
sketch "Sketch6" plane through (0, 2.54, 0) normal (0, 1, 0) x (1, 0, 0)
  line L0 (22.4402, 31.1118) -> (31.5374, 30.5468) projected
  line L1 (31.5374, 30.5468) -> (24.5097, 24.7424) projected
  line L2 (24.5097, 24.7424) -> (26.7836, 15.9159) projected
  line L3 (26.7836, 15.9159) -> (19.0916, 20.806) projected
  line L4 (19.0916, 20.806) -> (11.3997, 15.9159) projected
  line L5 (11.3997, 15.9159) -> (13.6736, 24.7424) projected
  line L6 (13.6736, 24.7424) -> (6.6459, 30.5468) projected
  line L7 (6.6459, 30.5468) -> (15.7431, 31.1118) projected
  line L8 (15.7431, 31.1118) -> (19.0916, 39.5891) projected
  line L9 (19.0916, 39.5891) -> (22.4402, 31.1118) projected
  line L10 (-16.7308, 13.6918) -> (-27.8255, 20.0974) projected
  line L11 (-27.8255, 20.0974) -> (-27.8255, 32.9084) projected
  line L12 (-27.8255, 32.9084) -> (-16.7308, 39.3139) projected
  line L13 (-16.7308, 39.3139) -> (-5.6361, 32.9084) projected
  line L14 (-5.6361, 32.9084) -> (-5.6361, 20.0974) projected
  line L15 (-5.6361, 20.0974) -> (-16.7308, 13.6918) projected
  circle A0 centre (0, 0) radius 50.8 projected
  line L16 (22.0447, 4.397) -> (22.0447, 5.9805) projected
  line L17 (22.0447, 5.9805) -> (31.5841, 5.9805) projected
  line L18 (31.5841, 5.9805) -> (32.8893, 2.3625) projected
  line L19 (32.8893, 2.3625) -> (31.4017, 1.825) projected
  line L20 (27.9852, 4.1475) -> (26.2386, 4.1475) projected
  line L21 (26.2386, 4.1475) -> (26.2386, 1.2972) projected
  line L22 (26.2386, 1.2972) -> (26.8144, 1.2972) projected
  line L23 (28.11, 2.4872) -> (28.11, 2.9191) projected
  line L24 (28.11, 2.9191) -> (29.5687, 2.9191) projected
  line L25 (29.5687, 2.9191) -> (29.5687, -1.9178) projected
  line L26 (29.5687, -1.9178) -> (28.11, -1.9178) projected
  line L27 (28.11, -1.9178) -> (28.11, -1.4283) projected
  line L28 (26.7568, -0.2959) -> (26.2386, -0.2959) projected
  line L29 (26.2386, -0.2959) -> (26.2386, -2.9159) projected
  line L30 (26.9487, -3.6164) -> (27.9084, -3.6164) projected
  line L31 (31.9296, -0.6894) -> (33.4267, -1.198) projected
  line L32 (33.4267, -1.198) -> (31.9296, -5.4495) projected
  line L33 (31.9296, -5.4495) -> (22.0447, -5.4495) projected
  line L34 (22.0447, -5.4495) -> (22.0447, -3.866) projected
  line L35 (22.0447, -3.866) -> (22.3326, -3.866) projected
  line L36 (23.4171, -2.8007) -> (23.4171, 3.4181) projected
  line L37 (22.5533, 4.397) -> (22.0447, 4.397) projected
  line L38 (-2.1013, 4.397) -> (-2.1013, 5.9805) projected
  line L39 (-2.1013, 5.9805) -> (2.5244, 5.9805) projected
  line L40 (2.5244, 5.9805) -> (5.8834, -0.6894) projected
  line L41 (5.8834, -0.6894) -> (5.8834, 3.3893) projected
  line L42 (5.0676, 4.397) -> (4.511, 4.397) projected
  line L43 (4.511, 4.397) -> (4.511, 5.9805) projected
  line L44 (4.511, 5.9805) -> (9.2135, 5.9805) projected
  line L45 (9.2135, 5.9805) -> (9.2135, 4.397) projected
  line L46 (9.2135, 4.397) -> (8.6953, 4.397) projected
  line L47 (7.8412, 3.3893) -> (7.8412, -5.4495) projected
  line L48 (7.8412, -5.4495) -> (5.4899, -5.4495) projected
  line L49 (5.4899, -5.4495) -> (1.248, 2.9767) projected
  line L50 (1.248, 2.9767) -> (1.248, -2.9159) projected
  line L51 (2.0734, -3.866) -> (2.6204, -3.866) projected
  line L52 (2.6204, -3.866) -> (2.6204, -5.4495) projected
  line L53 (2.6204, -5.4495) -> (-2.1013, -5.4495) projected
  line L54 (-2.1013, -5.4495) -> (-2.1013, -3.866) projected
  line L55 (-2.1013, -3.866) -> (-1.6119, -3.866) projected
  line L56 (-0.7289, -3.0406) -> (-0.7289, 3.5141) projected
  line L57 (-1.4967, 4.397) -> (-2.1013, 4.397) projected
  line L58 (-45.4605, 4.397) -> (-45.4605, 5.9805) projected
  line L59 (-45.4605, 5.9805) -> (-39.8942, 5.9805) projected
  line L60 (-39.8942, 5.9805) -> (-39.8942, 4.397) projected
  line L61 (-39.8942, 4.397) -> (-40.4028, 4.397) projected
  line L62 (-41.2666, 3.4277) -> (-41.2666, -2.8871) projected
  line L63 (-40.4988, -3.866) -> (-39.8942, -3.866) projected
  line L64 (-39.8942, -3.866) -> (-39.8942, -5.4495) projected
  line L65 (-39.8942, -5.4495) -> (-45.4605, -5.4495) projected
  line L66 (-45.4605, -5.4495) -> (-45.4605, -3.866) projected
  line L67 (-45.4605, -3.866) -> (-45.0094, -3.866) projected
  line L68 (-44.0881, -2.9734) -> (-44.0881, 3.3702) projected
  line L69 (-44.9518, 4.397) -> (-45.4605, 4.397) projected
  line L70 (-32.946, 4.397) -> (-32.946, 5.9805) projected
  line L71 (-32.946, 5.9805) -> (-26.9095, 5.9805) projected
  line L72 (-26.8039, -0.9197) -> (-28.7521, -0.9197) projected
  line L73 (-28.7521, -0.9197) -> (-28.7521, -3.0598) projected
  line L74 (-27.9556, -3.866) -> (-27.3797, -3.866) projected
  line L75 (-27.3797, -3.866) -> (-27.3797, -5.4495) projected
  line L76 (-27.3797, -5.4495) -> (-32.946, -5.4495) projected
  line L77 (-32.946, -5.4495) -> (-32.946, -3.866) projected
  line L78 (-32.946, -3.866) -> (-32.5621, -3.866) projected
  line L79 (-31.5736, -2.8967) -> (-31.5736, 3.3798) projected
  line L80 (-32.399, 4.397) -> (-32.946, 4.397) projected
  line L81 (-21.9383, 4.349) -> (-21.9383, 5.9805) projected
  line L82 (-21.9383, 5.9805) -> (-14.8941, 5.9805) projected
  line L83 (-13.7041, -0.3439) -> (-11.3528, -3.079) projected
  line L84 (-11.3528, -3.079) -> (-11.2568, -3.2038) projected
  line L85 (-9.9324, -3.866) -> (-9.443, -3.866) projected
  line L86 (-9.443, -3.866) -> (-9.443, -5.4495) projected
  line L87 (-9.443, -5.4495) -> (-13.109, -5.4495) projected
  line L88 (-13.109, -5.4495) -> (-16.7751, -0.5262) projected
  line L89 (-16.7751, -0.5262) -> (-17.7252, -0.5262) projected
  line L90 (-17.7252, -0.5262) -> (-17.7252, -2.8007) projected
  line L91 (-16.8711, -3.866) -> (-16.3528, -3.866) projected
  line L92 (-16.3528, -3.866) -> (-16.3528, -5.4495) projected
  line L93 (-16.3528, -5.4495) -> (-21.9383, -5.4495) projected
  line L94 (-21.9383, -5.4495) -> (-21.9383, -3.866) projected
  line L95 (-21.9383, -3.866) -> (-21.4296, -3.866) projected
  line L96 (-20.5659, -2.9063) -> (-20.5659, 3.5237) projected
  line L97 (-21.2761, 4.3586) -> (-21.5064, 4.349) projected
  line L98 (-21.5064, 4.349) -> (-21.9383, 4.349) projected
  line L99 (-8.896, 4.397) -> (-8.896, 5.9805) projected
  line L100 (-8.896, 5.9805) -> (-3.3297, 5.9805) projected
  line L101 (-3.3297, 5.9805) -> (-3.3297, 4.397) projected
  line L102 (-3.3297, 4.397) -> (-3.8384, 4.397) projected
  line L103 (-4.7021, 3.4277) -> (-4.7021, -2.8871) projected
  line L104 (-3.9343, -3.866) -> (-3.3297, -3.866) projected
  line L105 (-3.3297, -3.866) -> (-3.3297, -5.4495) projected
  line L106 (-3.3297, -5.4495) -> (-8.896, -5.4495) projected
  line L107 (-8.896, -5.4495) -> (-8.896, -3.866) projected
  line L108 (-8.896, -3.866) -> (-8.4449, -3.866) projected
  line L109 (-7.5236, -2.9734) -> (-7.5236, 3.3702) projected
  line L110 (-8.3873, 4.397) -> (-8.896, 4.397) projected
  line L111 (9.6742, 2.3529) -> (11.0849, 6.3644) projected
  line L112 (11.0849, 6.3644) -> (12.1598, 6.3644) projected
  line L113 (12.1598, 6.3644) -> (12.275, 5.9805) projected
  line L114 (12.275, 5.9805) -> (18.7241, 5.9805) projected
  line L115 (18.7241, 5.9805) -> (18.8585, 6.3644) projected
  line L116 (18.8585, 6.3644) -> (19.9429, 6.3644) projected
  line L117 (19.9429, 6.3644) -> (21.3633, 2.3529) projected
  line L118 (21.3633, 2.3529) -> (19.8374, 1.825) projected
  line L119 (16.9199, 3.802) -> (16.9199, -2.7623) projected
  line L120 (18.2923, -3.866) -> (18.2923, -5.4495) projected
  line L121 (18.2923, -5.4495) -> (12.726, -5.4495) projected
  line L122 (12.726, -5.4495) -> (12.726, -3.866) projected
  line L123 (12.726, -3.866) -> (13.0619, -3.866) projected
  line L124 (14.0984, -2.8199) -> (14.0984, 3.898) projected
  line L125 (11.1713, 1.825) -> (9.6742, 2.3529) projected
  line L126 (34.0985, 4.397) -> (34.0985, 5.9805) projected
  line L127 (34.0985, 5.9805) -> (40.087, 5.9805) projected
  line L128 (39.3768, -5.4495) -> (34.0985, -5.4495) projected
  line L129 (34.0985, -5.4495) -> (34.0985, -3.866) projected
  line L130 (34.0985, -3.866) -> (34.492, -3.866) projected
  line L131 (35.4709, -2.8295) -> (35.4709, 3.4181) projected
  line L132 (34.492, 4.397) -> (34.0985, 4.397) projected
  line L133 (-11.1834, 16.8946) -> (-22.2781, 36.1112) construction
  line L134 (-11.1834, 36.1112) -> (-22.2781, 16.8946) construction
  line L135 (-27.8255, 32.9084) -> (-16.7308, 26.5029)
  line L136 (-5.6361, 32.9084) -> (-16.7308, 26.5029)
  constraints: 8 end point, 5 midpoint, 1 perpendicular, 55 other
extrude "Extrusion5" add sketch "Sketch6" against normal blind 2.54 separate body contours L12 L13 L136 L135
sketch "Sketch7" plane through (0, 2.54, 0) normal (0, 1, 0) x (1, 0, 0)
  line L0 (-16.7308, 39.3139) -> (-27.8255, 32.9084) projected
  line L1 (-27.8255, 32.9084) -> (-16.7308, 26.5029) projected
  line L2 (-16.7308, 26.5029) -> (-5.6361, 32.9084) projected
  line L3 (-5.6361, 32.9084) -> (-16.7308, 39.3139) projected
  line L4 (-5.6361, 20.0974) -> (-16.7308, 13.6918) projected
  line L5 (-16.7308, 26.5029) -> (-16.7308, 13.6918)
  line L6 (-16.7308, 13.6918) -> (-5.6361, 20.0974)
  line L7 (-5.6361, 20.0974) -> (-5.6361, 32.9084)
  line L8 (-5.6361, 32.9084) -> (-16.7308, 26.5029)
  point P0 (0, 0)
  constraints: 8 end point, 2 equal length, 1 vertical
extrude "Extrusion6" add sketch "Sketch7" against normal blind 2.54 separate body contours L7 L4 L5 L2
sketch "Sketch8" plane through (0, 2.54, 0) normal (0, 1, 0) x (1, 0, 0)
  line L0 (-16.7308, 39.3139) -> (-27.8255, 32.9084) projected
  line L1 (-27.8255, 32.9084) -> (-16.7308, 26.5029) projected
  line L2 (-16.7308, 26.5029) -> (-5.6361, 32.9084) projected
  line L3 (-5.6361, 32.9084) -> (-16.7308, 39.3139) projected
  line L4 (-16.7308, 13.6918) -> (-5.6361, 20.0974) projected
  line L5 (-5.6361, 20.0974) -> (-5.6361, 32.9084) projected
  line L6 (-5.6361, 32.9084) -> (-16.7308, 26.5029) projected
  line L7 (-16.7308, 26.5029) -> (-16.7308, 13.6918) projected
  line L8 (22.4402, 31.1118) -> (31.5374, 30.5468) projected
  line L9 (31.5374, 30.5468) -> (24.5097, 24.7424) projected
  line L10 (24.5097, 24.7424) -> (26.7836, 15.9159) projected
  line L11 (26.7836, 15.9159) -> (19.0916, 20.806) projected
  line L12 (19.0916, 20.806) -> (11.3997, 15.9159) projected
  line L13 (11.3997, 15.9159) -> (13.6736, 24.7424) projected
  line L14 (13.6736, 24.7424) -> (6.6459, 30.5468) projected
  line L15 (6.6459, 30.5468) -> (15.7431, 31.1118) projected
  line L16 (15.7431, 31.1118) -> (19.0916, 39.5891) projected
  line L17 (19.0916, 39.5891) -> (22.4402, 31.1118) projected
  line L18 (-16.7308, 13.6918) -> (-27.8255, 20.0974) projected
  line L19 (-27.8255, 20.0974) -> (-27.8255, 32.9084) projected
  line L20 (-27.8255, 32.9084) -> (-16.7308, 39.3139) projected
  line L21 (-16.7308, 39.3139) -> (-5.6361, 32.9084) projected
  line L22 (-5.6361, 32.9084) -> (-5.6361, 20.0974) projected
  line L23 (-5.6361, 20.0974) -> (-16.7308, 13.6918) projected
  circle A0 centre (0, 0) radius 50.8 projected
  line L24 (22.0447, 4.397) -> (22.0447, 5.9805) projected
  line L25 (22.0447, 5.9805) -> (31.5841, 5.9805) projected
  line L26 (31.5841, 5.9805) -> (32.8893, 2.3625) projected
  line L27 (32.8893, 2.3625) -> (31.4017, 1.825) projected
  line L28 (27.9852, 4.1475) -> (26.2386, 4.1475) projected
  line L29 (26.2386, 4.1475) -> (26.2386, 1.2972) projected
  line L30 (26.2386, 1.2972) -> (26.8144, 1.2972) projected
  line L31 (28.11, 2.4872) -> (28.11, 2.9191) projected
  line L32 (28.11, 2.9191) -> (29.5687, 2.9191) projected
  line L33 (29.5687, 2.9191) -> (29.5687, -1.9178) projected
  line L34 (29.5687, -1.9178) -> (28.11, -1.9178) projected
  line L35 (28.11, -1.9178) -> (28.11, -1.4283) projected
  line L36 (26.7568, -0.2959) -> (26.2386, -0.2959) projected
  line L37 (26.2386, -0.2959) -> (26.2386, -2.9159) projected
  line L38 (26.9487, -3.6164) -> (27.9084, -3.6164) projected
  line L39 (31.9296, -0.6894) -> (33.4267, -1.198) projected
  line L40 (33.4267, -1.198) -> (31.9296, -5.4495) projected
  line L41 (31.9296, -5.4495) -> (22.0447, -5.4495) projected
  line L42 (22.0447, -5.4495) -> (22.0447, -3.866) projected
  line L43 (22.0447, -3.866) -> (22.3326, -3.866) projected
  line L44 (23.4171, -2.8007) -> (23.4171, 3.4181) projected
  line L45 (22.5533, 4.397) -> (22.0447, 4.397) projected
  line L46 (-2.1013, 4.397) -> (-2.1013, 5.9805) projected
  line L47 (-2.1013, 5.9805) -> (2.5244, 5.9805) projected
  line L48 (2.5244, 5.9805) -> (5.8834, -0.6894) projected
  line L49 (5.8834, -0.6894) -> (5.8834, 3.3893) projected
  line L50 (5.0676, 4.397) -> (4.511, 4.397) projected
  line L51 (4.511, 4.397) -> (4.511, 5.9805) projected
  line L52 (4.511, 5.9805) -> (9.2135, 5.9805) projected
  line L53 (9.2135, 5.9805) -> (9.2135, 4.397) projected
  line L54 (9.2135, 4.397) -> (8.6953, 4.397) projected
  line L55 (7.8412, 3.3893) -> (7.8412, -5.4495) projected
  line L56 (7.8412, -5.4495) -> (5.4899, -5.4495) projected
  line L57 (5.4899, -5.4495) -> (1.248, 2.9767) projected
  line L58 (1.248, 2.9767) -> (1.248, -2.9159) projected
  line L59 (2.0734, -3.866) -> (2.6204, -3.866) projected
  line L60 (2.6204, -3.866) -> (2.6204, -5.4495) projected
  line L61 (2.6204, -5.4495) -> (-2.1013, -5.4495) projected
  line L62 (-2.1013, -5.4495) -> (-2.1013, -3.866) projected
  line L63 (-2.1013, -3.866) -> (-1.6119, -3.866) projected
  line L64 (-0.7289, -3.0406) -> (-0.7289, 3.5141) projected
  line L65 (-1.4967, 4.397) -> (-2.1013, 4.397) projected
  line L66 (-45.4605, 4.397) -> (-45.4605, 5.9805) projected
  line L67 (-45.4605, 5.9805) -> (-39.8942, 5.9805) projected
  line L68 (-39.8942, 5.9805) -> (-39.8942, 4.397) projected
  line L69 (-39.8942, 4.397) -> (-40.4028, 4.397) projected
  line L70 (-41.2666, 3.4277) -> (-41.2666, -2.8871) projected
  line L71 (-40.4988, -3.866) -> (-39.8942, -3.866) projected
  line L72 (-39.8942, -3.866) -> (-39.8942, -5.4495) projected
  line L73 (-39.8942, -5.4495) -> (-45.4605, -5.4495) projected
  line L74 (-45.4605, -5.4495) -> (-45.4605, -3.866) projected
  line L75 (-45.4605, -3.866) -> (-45.0094, -3.866) projected
  line L76 (-44.0881, -2.9734) -> (-44.0881, 3.3702) projected
  line L77 (-44.9518, 4.397) -> (-45.4605, 4.397) projected
  line L78 (-32.946, 4.397) -> (-32.946, 5.9805) projected
  line L79 (-32.946, 5.9805) -> (-26.9095, 5.9805) projected
  line L80 (-26.8039, -0.9197) -> (-28.7521, -0.9197) projected
  line L81 (-28.7521, -0.9197) -> (-28.7521, -3.0598) projected
  line L82 (-27.9556, -3.866) -> (-27.3797, -3.866) projected
  line L83 (-27.3797, -3.866) -> (-27.3797, -5.4495) projected
  line L84 (-27.3797, -5.4495) -> (-32.946, -5.4495) projected
  line L85 (-32.946, -5.4495) -> (-32.946, -3.866) projected
  line L86 (-32.946, -3.866) -> (-32.5621, -3.866) projected
  line L87 (-31.5736, -2.8967) -> (-31.5736, 3.3798) projected
  line L88 (-32.399, 4.397) -> (-32.946, 4.397) projected
  line L89 (-21.9383, 4.349) -> (-21.9383, 5.9805) projected
  line L90 (-21.9383, 5.9805) -> (-14.8941, 5.9805) projected
  line L91 (-13.7041, -0.3439) -> (-11.3528, -3.079) projected
  line L92 (-11.3528, -3.079) -> (-11.2568, -3.2038) projected
  line L93 (-9.9324, -3.866) -> (-9.443, -3.866) projected
  line L94 (-9.443, -3.866) -> (-9.443, -5.4495) projected
  line L95 (-9.443, -5.4495) -> (-13.109, -5.4495) projected
  line L96 (-13.109, -5.4495) -> (-16.7751, -0.5262) projected
  line L97 (-16.7751, -0.5262) -> (-17.7252, -0.5262) projected
  line L98 (-17.7252, -0.5262) -> (-17.7252, -2.8007) projected
  line L99 (-16.8711, -3.866) -> (-16.3528, -3.866) projected
  line L100 (-16.3528, -3.866) -> (-16.3528, -5.4495) projected
  line L101 (-16.3528, -5.4495) -> (-21.9383, -5.4495) projected
  line L102 (-21.9383, -5.4495) -> (-21.9383, -3.866) projected
  line L103 (-21.9383, -3.866) -> (-21.4296, -3.866) projected
  line L104 (-20.5659, -2.9063) -> (-20.5659, 3.5237) projected
  line L105 (-21.2761, 4.3586) -> (-21.5064, 4.349) projected
  line L106 (-21.5064, 4.349) -> (-21.9383, 4.349) projected
  line L107 (-8.896, 4.397) -> (-8.896, 5.9805) projected
  line L108 (-8.896, 5.9805) -> (-3.3297, 5.9805) projected
  line L109 (-3.3297, 5.9805) -> (-3.3297, 4.397) projected
  line L110 (-3.3297, 4.397) -> (-3.8384, 4.397) projected
  line L111 (-4.7021, 3.4277) -> (-4.7021, -2.8871) projected
  line L112 (-3.9343, -3.866) -> (-3.3297, -3.866) projected
  line L113 (-3.3297, -3.866) -> (-3.3297, -5.4495) projected
  line L114 (-3.3297, -5.4495) -> (-8.896, -5.4495) projected
  line L115 (-8.896, -5.4495) -> (-8.896, -3.866) projected
  line L116 (-8.896, -3.866) -> (-8.4449, -3.866) projected
  line L117 (-7.5236, -2.9734) -> (-7.5236, 3.3702) projected
  line L118 (-8.3873, 4.397) -> (-8.896, 4.397) projected
  line L119 (9.6742, 2.3529) -> (11.0849, 6.3644) projected
  line L120 (11.0849, 6.3644) -> (12.1598, 6.3644) projected
  line L121 (12.1598, 6.3644) -> (12.275, 5.9805) projected
  line L122 (12.275, 5.9805) -> (18.7241, 5.9805) projected
  line L123 (18.7241, 5.9805) -> (18.8585, 6.3644) projected
  line L124 (18.8585, 6.3644) -> (19.9429, 6.3644) projected
  line L125 (19.9429, 6.3644) -> (21.3633, 2.3529) projected
  line L126 (21.3633, 2.3529) -> (19.8374, 1.825) projected
  line L127 (16.9199, 3.802) -> (16.9199, -2.7623) projected
  line L128 (18.2923, -3.866) -> (18.2923, -5.4495) projected
  line L129 (18.2923, -5.4495) -> (12.726, -5.4495) projected
  line L130 (12.726, -5.4495) -> (12.726, -3.866) projected
  line L131 (12.726, -3.866) -> (13.0619, -3.866) projected
  line L132 (14.0984, -2.8199) -> (14.0984, 3.898) projected
  line L133 (11.1713, 1.825) -> (9.6742, 2.3529) projected
  line L134 (34.0985, 4.397) -> (34.0985, 5.9805) projected
  line L135 (34.0985, 5.9805) -> (40.087, 5.9805) projected
  line L136 (39.3768, -5.4495) -> (34.0985, -5.4495) projected
  line L137 (34.0985, -5.4495) -> (34.0985, -3.866) projected
  line L138 (34.0985, -3.866) -> (34.492, -3.866) projected
  line L139 (35.4709, -2.8295) -> (35.4709, 3.4181) projected
  line L140 (34.492, 4.397) -> (34.0985, 4.397) projected
  constraints: 55 other
extrude "Extrusion7" add sketch "Sketch8" against normal blind 2.54 separate body contours L1 L7 L18 L19